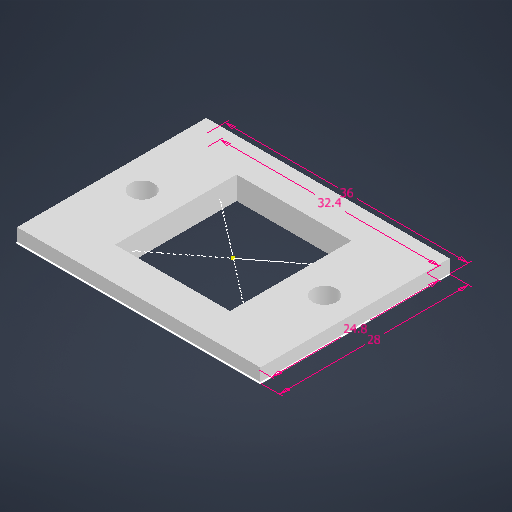
# Autodesk Inventor part: network panel
Saved by Autodesk Inventor 2026.2 (Build 302298010, 298A)
## iProperties
Created: 2026-09-22
Part Number: network panel
Material: Generic
Document SubType Name: Modeling
Designer: Graeme
Density: 1 g/cm^3
Appearance: Default
Author: Graeme
## iProperties of the stored document network panel_3DPrint.ipt
Created: 2026-09-22
Part Number: network panel_3DPrint
Material: Generic
Document SubType Name: Modeling
Designer: Graeme
Density: 1 g/cm^3
Appearance: Default
Author: Graeme
Autodesk Inventor part; units mm, degrees
ref_plane "YZ Plane" through (0, 0, 0) normal (1, 0, 0) x (0, 1, 0)
ref_plane "XZ Plane" through (0, 0, 0) normal (0, 1, 0) x (-1, 0, 0)
ref_plane "XY Plane" through (0, 0, 0) normal (0, 0, 1) x (1, 0, 0)
sketch "Sketch1" plane through (0, 0, 0) normal (0, 1, 0) x (-1, 0, 0)
  line L0 (16.2, 12.4) -> (-16.2, 12.4)
  line L1 (-16.2, 12.4) -> (-16.2, -12.4)
  line L2 (-16.2, -12.4) -> (16.2, -12.4)
  line L3 (16.2, -12.4) -> (16.2, 12.4)
  line L4 (16.2, 12.4) -> (-16.2, -12.4) construction
  line L5 (-16.2, 12.4) -> (16.2, -12.4) construction
  point P0 (0, 0)
  dimension "d0" = 32.4
  dimension "d1" = 24.8
  constraints: 12 end point, 2 midpoint, 2 parallel, 1 horizontal, 1 perpendicular
  measures "d0" distance of L2.end L1.end
  measures "d1" distance of L1.end L0.end
extrude "Extrusion1" add sketch "Sketch1" against normal blind 1.4
sketch "Sketch2" plane through (0, 0, 0) normal (0, 1, 0) x (1, 0, 0)
  line L0 (-18, -14) -> (18, -14)
  line L1 (18, -14) -> (18, 14)
  line L2 (18, 14) -> (-18, 14)
  line L3 (-18, 14) -> (-18, -14)
  line L4 (-18, -14) -> (18, 14) construction
  line L5 (18, -14) -> (-18, 14) construction
  point P0 (0, 0)
  dimension "d4" = 36
  dimension "d5" = 28
  constraints: 12 end point, 2 midpoint, 2 parallel, 1 horizontal, 1 perpendicular
  measures "d4" distance of L2.end L1.end
  measures "d5" distance of L1.end L0.end
extrude "Extrusion2" add sketch "Sketch2" along normal blind 2
sketch "Sketch3" plane through (0, 2, 0) normal (0, 1, 0) x (1, 0, 0)
  line L0 (-8.5, -9) -> (8.5, -9)
  line L1 (8.5, -9) -> (8.5, 9)
  line L2 (8.5, 9) -> (-8.5, 9)
  line L3 (-8.5, 9) -> (-8.5, -9)
  line L4 (-8.5, -9) -> (8.5, 9) construction
  line L5 (8.5, -9) -> (-8.5, 9) construction
  circle A0 centre (-13.5, 0) radius 1.75
  circle A1 centre (13.5, 0) radius 1.75
  point P0 (0, 0)
  dimension "d8" = 17
  dimension "d9" = 18
  dimension "d10" = 13.5
  dimension "d11" = 13.5
  dimension "d12" = 3.5
  dimension "d13" = 3.5
  constraints: 12 end point, 2 centre point, 2 coincident, 2 midpoint, 2 parallel, 1 horizontal, 1 perpendicular
  measures "d8" distance of L2.end L1.end
  measures "d9" distance of L1.end L0.end
  measures "d10" distance of point (0, 0) point (-13.5, 0)
  measures "d11" distance of point (13.5, 0) point (0, 0)
  measures "d12" diameter of A0
  measures "d13" diameter of A1
extrude "Extrusion3" cut sketch "Sketch3" against normal up to surface (3.4 mm away)
equation "\"d11\" = d10"
body "Solid1"
